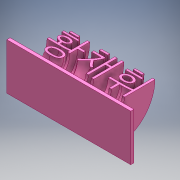
# Autodesk Inventor part: 이름
Saved by Autodesk Inventor 2016 (Build 200138000, 138)
## iProperties
Created: 2024-03-15
Part Number: 이름
Material: 일반
Document SubType Name: Modeling
Designer: pc
Density: 1 g/cm^3
Appearance: 분홍색
Author: pc
Autodesk Inventor part; units mm, degrees
ref_plane "YZ Plane" through (0, 0, 0) normal (1, 0, 0) x (0, 1, 0)
ref_plane "XZ Plane" through (0, 0, 0) normal (0, 1, 0) x (-1, 0, 0)
ref_plane "XY Plane" through (0, 0, 0) normal (0, 0, 1) x (1, 0, 0)
sketch "스케치1" plane through (0, 0, 0) normal (0, 0, 1) x (1, 0, 0)
  line L0 (-57.8923, 18.2462) -> (64.5553, 18.2462) construction
  line L1 (64.5553, 18.2462) -> (64.5553, -22.5955) construction
  line L2 (64.5553, -22.5955) -> (-57.8923, -22.5955) construction
  line L3 (-57.8923, -22.5955) -> (-57.8923, 18.2462) construction
  line L4 (-61.4665, -6.0943) -> (4.51, -6.0943)
  line L5 (-57.0918, 6.7107) -> (-57.0918, 8.0362)
  line L6 (-57.0918, 8.0362) -> (-51.7768, 8.0362)
  line L7 (-51.7768, 8.0362) -> (-51.7768, 9.3354)
  spline S0 degree 2 poles (-51.7768, 9.3354) (-53.1679, 9.4535) (-54.0734, 10.0441) knots 0 0 0 1 1 1
  spline S1 degree 2 poles (-54.0734, 10.0441) (-55.1889, 10.7659) (-55.1889, 12.8393) (-52.9317, 14.2829) (-51.0682, 14.2829) knots 0 0 0 1 2 3 3 3
  spline S2 degree 2 poles (-51.0682, 14.2829) (-49.2178, 14.2829) (-46.9606, 12.8393) (-46.9606, 11.8026) knots 0 0 0 1 2 2 2
  spline S3 degree 2 poles (-46.9606, 11.8026) (-46.9606, 10.7659) (-48.1023, 10.0441) knots 0 0 0 1 1 1
  spline S4 degree 2 poles (-48.1023, 10.0441) (-48.9684, 9.4798) (-50.2676, 9.3354) knots 0 0 0 1 1 1
  line L8 (-50.2676, 9.3354) -> (-50.2676, 8.0362)
  line L9 (-50.2676, 8.0362) -> (-47.8005, 8.0362)
  spline S5 degree 2 poles (-47.8005, 8.0362) (-47.1443, 8.0362) (-45.6351, 8.1018) (-44.1259, 8.2855) (-43.5222, 8.443) knots 0 0 0 1 2 3 3 3
  line L10 (-43.5222, 8.443) -> (-43.5222, 18.2199)
  line L11 (-43.5222, 18.2199) -> (-42.0393, 18.2199)
  line L12 (-42.0393, 18.2199) -> (-42.0393, 11.9995)
  line L13 (-42.0393, 11.9995) -> (-38.4041, 11.9995)
  line L14 (-38.4041, 11.9995) -> (-38.4041, 10.674)
  line L15 (-38.4041, 10.674) -> (-42.0393, 10.674)
  line L16 (-42.0393, 10.674) -> (-42.0393, 5.8446)
  line L17 (-42.0393, 5.8446) -> (-43.5222, 5.8446)
  line L18 (-43.5222, 5.8446) -> (-43.5222, 7.1307)
  spline S6 degree 2 poles (-43.5222, 7.1307) (-44.0865, 6.9995) (-45.5039, 6.8288) (-46.9999, 6.737) (-48.3648, 6.7107) (-48.8372, 6.7107) knots 0 0 0 1 2 3 4 4 4
  line L19 (-48.8372, 6.7107) -> (-57.0918, 6.7107)
  spline S7 degree 2 poles (-52.7217, 1.9601) (-52.7217, 3.6136) (-49.7033, 5.1622) (-47.3018, 5.1884) knots 0 0 0 1 2 2 2
  spline S8 degree 2 poles (-47.3018, 5.1884) (-44.9133, 5.1622) (-41.9343, 3.6136) (-41.9343, 1.9601) knots 0 0 0 1 2 2 2
  spline S9 degree 2 poles (-41.9343, 1.9601) (-41.9343, 0.2803) (-44.8083, -1.2026) (-47.3018, -1.2026) knots 0 0 0 1 2 2 2
  spline S10 degree 2 poles (-47.3018, -1.2026) (-49.8083, -1.2026) (-52.7217, 0.3065) (-52.7217, 1.9601) knots 0 0 0 1 2 2 2
  spline S11 degree 2 poles (-51.1863, 1.947) (-51.1863, 0.7396) (-48.9159, 0.0834) (-47.3018, 0.0834) knots 0 0 0 1 2 2 2
  spline S12 degree 2 poles (-47.3018, 0.0834) (-45.6876, 0.0834) (-43.4172, 0.7396) (-43.4172, 1.947) knots 0 0 0 1 2 2 2
  spline S13 degree 2 poles (-43.4172, 1.947) (-43.4435, 3.0624) (-45.6876, 3.9023) (-47.3018, 3.9023) knots 0 0 0 1 2 2 2
  spline S14 degree 2 poles (-47.3018, 3.9023) (-48.9159, 3.9023) (-51.2125, 2.9706) (-51.1863, 1.947) knots 0 0 0 1 2 2 2
  line L20 (-56.1207, 14.9391) -> (-56.1207, 16.1596)
  line L21 (-56.1207, 16.1596) -> (-46.1075, 16.1596)
  line L22 (-46.1075, 16.1596) -> (-46.1075, 14.9391)
  line L23 (-46.1075, 14.9391) -> (-56.1207, 14.9391)
  spline S15 degree 2 poles (-53.6928, 11.8026) (-53.6928, 11.2383) (-52.328, 10.5821) (-51.0682, 10.5821) knots 0 0 0 1 2 2 2
  spline S16 degree 2 poles (-51.0682, 10.5821) (-49.769, 10.5821) (-48.4435, 11.2383) (-48.4435, 11.8026) knots 0 0 0 1 2 2 2
  spline S17 degree 2 poles (-48.4435, 11.8026) (-48.4435, 12.3669) (-49.769, 13.0231) (-51.0682, 13.0231) knots 0 0 0 1 2 2 2
  spline S18 degree 2 poles (-51.0682, 13.0231) (-52.328, 13.0231) (-53.6928, 12.3669) (-53.6928, 11.8026) knots 0 0 0 1 2 2 2
  line L24 (-53.6797, 16.9995) -> (-53.6797, 18.2462)
  line L25 (-53.6797, 18.2462) -> (-48.1548, 18.2462)
  line L26 (-48.1548, 18.2462) -> (-48.1548, 16.9995)
  line L27 (-48.1548, 16.9995) -> (-53.6797, 16.9995)
  line L28 (-22.1705, 11.9863) -> (-22.1705, 18.1281)
  line L29 (-22.1705, 18.1281) -> (-20.6876, 18.1281)
  line L30 (-20.6876, 18.1281) -> (-20.6876, -0.6515)
  line L31 (-20.6876, -0.6515) -> (-22.1705, -0.6515)
  line L32 (-22.1705, -0.6515) -> (-22.1705, 10.6609)
  line L33 (-22.1705, 10.6609) -> (-24.7427, 10.6609)
  line L34 (-24.7427, 10.6609) -> (-24.7427, 0.0966)
  line L35 (-24.7427, 0.0966) -> (-26.2256, 0.0966)
  line L36 (-26.2256, 0.0966) -> (-26.2256, 18.0231)
  line L37 (-26.2256, 18.0231) -> (-24.7427, 18.0231)
  line L38 (-24.7427, 18.0231) -> (-24.7427, 11.9863)
  line L39 (-24.7427, 11.9863) -> (-22.1705, 11.9863)
  spline S19 degree 2 poles (-28.5747, 13.548) (-29.034, 12.4456) (-30.1495, 10.5034) (-30.8976, 9.4666) knots 0 0 0 1 2 2 2
  spline S20 degree 2 poles (-30.8976, 9.4666) (-30.1102, 8.3643) (-28.2729, 6.3564) (-27.2624, 5.6346) knots 0 0 0 1 2 2 2
  line L40 (-27.2624, 5.6346) -> (-28.1942, 4.6241)
  spline S21 degree 2 poles (-28.1942, 4.6241) (-29.0997, 5.3328) (-31.0157, 7.3144) (-31.8031, 8.3905) knots 0 0 0 1 2 2 2
  spline S22 degree 2 poles (-31.8031, 8.3905) (-32.7217, 7.2488) (-34.8083, 5.359) (-35.9763, 4.506) knots 0 0 0 1 2 2 2
  line L41 (-35.9763, 4.506) -> (-37.013, 5.5821)
  spline S23 degree 2 poles (-37.013, 5.5821) (-35.097, 6.6845) (-30.8976, 11.6189) (-30.2545, 13.3774) knots 0 0 0 1 2 2 2
  line L42 (-30.2545, 13.3774) -> (-36.0025, 13.3774)
  line L43 (-36.0025, 13.3774) -> (-36.0025, 14.716)
  line L44 (-36.0025, 14.716) -> (-28.5747, 14.716)
  line L45 (-28.5747, 14.716) -> (-28.5747, 13.548)
  line L46 (-34.6115, 16.6976) -> (-34.6115, 18.0231)
  spline S24 degree 2 poles (-34.6115, 18.0231) (-33.8634, 18.0231) (-31.9081, 18.0231) (-31.2256, 18.0231) knots 0 0 0 1 2 2 2
  line L47 (-31.2256, 18.0231) -> (-29.4015, 18.0231)
  line L48 (-29.4015, 18.0231) -> (-29.4015, 16.6976)
  line L49 (-29.4015, 16.6976) -> (-31.3044, 16.6976)
  spline S25 degree 2 poles (-31.3044, 16.6976) (-32.0524, 16.6976) (-33.9028, 16.6976) (-34.6115, 16.6976) knots 0 0 0 1 2 2 2
  line L50 (-9.8083, 4.5979) -> (-9.8083, -0.494)
  line L51 (-9.8083, -0.494) -> (-11.2913, -0.494)
  line L52 (-11.2913, -0.494) -> (-11.2913, 4.5979)
  line L53 (-11.2913, 4.5979) -> (-16.9606, 4.5979)
  line L54 (-16.9606, 4.5979) -> (-16.9606, 5.9233)
  line L55 (-16.9606, 5.9233) -> (-8.391, 5.9233)
  spline S26 degree 2 poles (-8.391, 5.9233) (-7.8529, 5.9233) (-6.4619, 5.9496) (-4.9789, 6.0283) (-3.5354, 6.1858) (-2.9317, 6.3564) knots 0 0 0 1 2 3 4 4 4
  line L56 (-2.9317, 6.3564) -> (-2.9317, 18.2199)
  line L57 (-2.9317, 18.2199) -> (-1.4619, 18.2199)
  line L58 (-1.4619, 18.2199) -> (-1.4619, -0.6515)
  line L59 (-1.4619, -0.6515) -> (-2.9317, -0.6515)
  line L60 (-2.9317, -0.6515) -> (-2.9317, 5.0178)
  spline S27 degree 2 poles (-2.9317, 5.0178) (-3.7322, 4.8079) (-6.6325, 4.5979) (-8.3648, 4.5979) knots 0 0 0 1 2 2 2
  line L61 (-8.3648, 4.5979) -> (-9.8083, 4.5979)
  spline S28 degree 2 poles (-14.9133, 10.2147) (-14.9133, 11.4745) (-12.4067, 13.2068) (-10.6088, 13.2068) knots 0 0 0 1 2 2 2
  spline S29 degree 2 poles (-10.6088, 13.2068) (-8.8109, 13.2068) (-6.2913, 11.4745) (-6.2913, 10.2147) knots 0 0 0 1 2 2 2
  spline S30 degree 2 poles (-6.2913, 10.2147) (-6.2913, 8.968) (-8.8109, 7.2357) (-10.6088, 7.2357) knots 0 0 0 1 2 2 2
  spline S31 degree 2 poles (-10.6088, 7.2357) (-12.4067, 7.2357) (-14.9133, 8.968) (-14.9133, 10.2147) knots 0 0 0 1 2 2 2
  spline S32 degree 2 poles (-13.4041, 10.2147) (-13.4041, 9.506) (-11.8162, 8.5349) (-10.6088, 8.5349) knots 0 0 0 1 2 2 2
  spline S33 degree 2 poles (-10.6088, 8.5349) (-9.3884, 8.5349) (-7.8005, 9.506) (-7.8005, 10.2147) knots 0 0 0 1 2 2 2
  spline S34 degree 2 poles (-7.8005, 10.2147) (-7.8005, 10.9102) (-9.3884, 11.9076) (-10.6088, 11.9076) knots 0 0 0 1 2 2 2
  spline S35 degree 2 poles (-10.6088, 11.9076) (-11.8162, 11.9076) (-13.4041, 10.9102) (-13.4041, 10.2147) knots 0 0 0 1 2 2 2
  line L62 (-5.7795, 14.1779) -> (-15.8057, 14.1779)
  line L63 (-15.8057, 14.1779) -> (-15.8057, 15.4771)
  line L64 (-15.8057, 15.4771) -> (-5.7795, 15.4771)
  line L65 (-5.7795, 15.4771) -> (-5.7795, 14.1779)
  line L66 (-13.5747, 16.7632) -> (-13.5747, 18.0624)
  spline S36 degree 2 poles (-13.5747, 18.0624) (-12.8267, 18.0624) (-11.055, 18.0624) (-10.3726, 18.0624) knots 0 0 0 1 2 2 2
  line L67 (-10.3726, 18.0624) -> (-8.0498, 18.0624)
  line L68 (-8.0498, 18.0624) -> (-8.0498, 16.7632)
  line L69 (-8.0498, 16.7632) -> (-10.4514, 16.7632)
  spline S37 degree 2 poles (-10.4514, 16.7632) (-11.1994, 16.7632) (-12.8923, 16.7632) (-13.5747, 16.7632) knots 0 0 0 1 2 2 2
  point P0 (0, 0)
  constraints: 2 end point, 1 horizontal, 2 other
revolve "회전1" add sketch "스케치1" angle 90 about axis through (-61.4665, -6.0943, 0) along (-1, 0, 0)
sketch "스케치2" plane through (-36.0025, -6.0943, -20.8103) normal (0, -1, 0) x (1, 0, 0)
  line L0 (45.8142, -6.3485) -> (-31.2888, -6.3485)
  line L1 (-31.2888, -6.3485) -> (-31.2888, 22.5651)
  line L2 (-31.2888, 22.5651) -> (45.8142, 22.5651)
  line L3 (45.8142, 22.5651) -> (45.8142, -6.3485)
  line L4 (45.8142, -6.3485) -> (-31.2888, 22.5651) construction
  line L5 (-31.2888, -6.3485) -> (45.8142, 22.5651) construction
  point P0 (36.0025, 20.8103)
  point P1 (7.2627, 8.1083)
  constraints: 12 end point, 2 midpoint, 2 parallel, 1 horizontal, 1 perpendicular
extrude "돌출1" add sketch "스케치2" along normal blind 2
